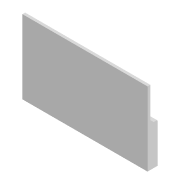
# Autodesk Inventor part: Display_A
Saved by Autodesk Inventor 2020 (Build 240168000, 168)
## iProperties
Created: 2021-10-24
Part Number: Display_A
Material: 一般
Document SubType Name: Modeling
Designer: ken113
Density: 1 g/cm^3
Appearance: 既定
Author: ken113
Autodesk Inventor part; units mm, degrees
ref_plane "YZ Plane" through (0, 0, 0) normal (1, 0, 0) x (0, 1, 0)
ref_plane "XZ Plane" through (0, 0, 0) normal (0, 1, 0) x (-1, 0, 0)
ref_plane "XY Plane" through (0, 0, 0) normal (0, 0, 1) x (1, 0, 0)
sketch "スケッチ1" plane through (0, 0, 0) normal (0, 0, 1) x (1, 0, 0)
  line L0 (369, -217.5) -> (-369, -217.5)
  line L1 (-369, -217.5) -> (-369, 217.5)
  line L2 (-369, 217.5) -> (369, 217.5)
  line L3 (369, 217.5) -> (369, -217.5)
  line L4 (369, -217.5) -> (-369, 217.5) construction
  line L5 (-369, -217.5) -> (369, 217.5) construction
  point P0 (0, 0)
  dimension "d0" = 738
  dimension "d1" = 435
  constraints: 12 end point, 2 midpoint, 2 parallel, 1 horizontal, 1 perpendicular
  measures "d0" distance of L1.end L2.end
  measures "d1" distance of L0.end L1.end
extrude "押し出し1" add sketch "スケッチ1" along normal blind 59
sketch "スケッチ2" plane through (369, -217.5, 0) normal (1, 0, 0) x (0, 0, -1)
  line L0 (0, 435) -> (-59, 435) projected
  line L1 (-42.8, 435) -> (0, 435)
  line L2 (0, 435) -> (0, 235)
  line L3 (0, 235) -> (-42.8, 235)
  line L4 (-42.8, 235) -> (-42.8, 435)
  line L5 (-59, 0) -> (-59, 435) projected
  point P0 (0, 217.5)
  dimension "d4" = 16.2
  dimension "d5" = 200
  constraints: 8 end point, 2 parallel, 1 horizontal, 1 perpendicular, 1 point on line
  measures "d4" distance between parallel lines of L4 L5
  measures "d5" distance between parallel lines of L0 L3
extrude "押し出し2" cut sketch "スケッチ2" against normal through all
chamfer "面取り1" distance 20 angle 45 1 edges at (0, 17.5, 42.8)
fillet "フィレット1" radius 5 3 edges at (0, 37.5, 42.8) (0, 17.5, 22.8) (0, 17.5, 0)
